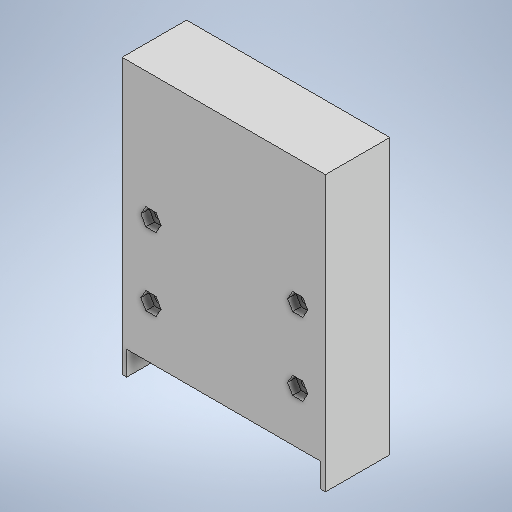
# Autodesk Inventor part: TES_Controller_V1_Case_Top
Saved by Autodesk Inventor 2025 (Build 290162000, 162)
## iProperties
Created: 2025-08-31
Part Number: TES_Controller_V1_Case_Top
Material: 常规
Document SubType Name: Modeling
Designer: 95052
Density: 1 g/cm^3
Appearance: 默认
Author: 95052
Autodesk Inventor part; units mm, degrees
ref_plane "YZ Plane" through (0, 0, 0) normal (1, 0, 0) x (0, 1, 0)
ref_plane "XZ Plane" through (0, 0, 0) normal (0, 1, 0) x (-1, 0, 0)
ref_plane "XY Plane" through (0, 0, 0) normal (0, 0, 1) x (1, 0, 0)
sketch "草图1" plane through (0, 0, 0) normal (0, 0, 1) x (1, 0, 0)
  line L0 (33.589, -45.4) -> (-33.589, -45.4)
  line L1 (-33.589, -45.4) -> (-33.589, 45.4)
  line L2 (-33.589, 45.4) -> (33.589, 45.4)
  line L3 (33.589, 45.4) -> (33.589, -45.4)
  line L4 (33.589, -45.4) -> (-33.589, 45.4) construction
  line L5 (-33.589, -45.4) -> (33.589, 45.4) construction
  line L6 (24.428, -20.313) -> (-24.072, -20.313) construction
  line L7 (-24.072, -20.313) -> (-24.072, 3.687) construction
  line L8 (-24.072, 3.687) -> (24.428, 3.687) construction
  line L9 (24.428, 3.687) -> (24.428, -20.313) construction
  line L10 (-22.3977, 6.587) -> (-20.7234, 3.687)
  line L11 (-20.7234, 3.687) -> (-22.3977, 0.787)
  line L12 (-22.3977, 0.787) -> (-25.7463, 0.787)
  line L13 (-25.7463, 0.787) -> (-27.4206, 3.687)
  line L14 (-27.4206, 3.687) -> (-25.7463, 6.587)
  line L15 (-25.7463, 6.587) -> (-22.3977, 6.587)
  line L16 (-22.3977, -17.413) -> (-20.7234, -20.313)
  line L17 (-20.7234, -20.313) -> (-22.3977, -23.213)
  line L18 (-22.3977, -23.213) -> (-25.7463, -23.213)
  line L19 (-25.7463, -23.213) -> (-27.4206, -20.313)
  line L20 (-27.4206, -20.313) -> (-25.7463, -17.413)
  line L21 (-25.7463, -17.413) -> (-22.3977, -17.413)
  line L22 (26.1023, -17.413) -> (27.7766, -20.313)
  line L23 (27.7766, -20.313) -> (26.1023, -23.213)
  line L24 (26.1023, -23.213) -> (22.7537, -23.213)
  line L25 (22.7537, -23.213) -> (21.0794, -20.313)
  line L26 (21.0794, -20.313) -> (22.7537, -17.413)
  line L27 (22.7537, -17.413) -> (26.1023, -17.413)
  line L28 (22.7537, 0.787) -> (21.0794, 3.687)
  line L29 (21.0794, 3.687) -> (22.7537, 6.587)
  line L30 (22.7537, 6.587) -> (26.1023, 6.587)
  line L31 (26.1023, 6.587) -> (27.7766, 3.687)
  line L32 (27.7766, 3.687) -> (26.1023, 0.787)
  line L33 (26.1023, 0.787) -> (22.7537, 0.787)
  point P0 (0, 0)
  point P1 (-24.072, -17.413)
  point P2 (24.428, -17.413)
  point P3 (24.428, 0.787)
  point P4 (24.428, 6.587)
  dimension "d0" = 90.8
  dimension "d1" = 67.178
  dimension "d2" = 25.087
  dimension "d3" = 9.161
  dimension "d4" = 9.517
  dimension "d5" = 41.713
  dimension "d6" = 2.9
  dimension "d7" = 2.9
  dimension "d8" = 2.9
  dimension "d9" = 2.9
  constraints: 68 end point, 6 midpoint, 4 coincident, 4 parallel, 3 point on line, 2 horizontal, 2 perpendicular, 52 other
  measures "d0" distance of L0.end L1.end
  measures "d1" distance of L0.start L0.end
  measures "d2" distance between parallel lines of L0 L6
  measures "d3" distance between parallel lines of L3 L9
  measures "d4" distance between parallel lines of L1 L7
  measures "d5" distance between parallel lines of L8 L2
  measures "d6" distance from line of L15 L7.end
  measures "d7" distance from line of L21 L6.end
  measures "d8" distance from line of L27 L6.start
  measures "d9" distance of point (24.428, 6.587) L8.end
extrude "拉伸1" add sketch "草图1" along normal blind 2
sketch "草图2" plane through (0, 0, 0) normal (0, 0, -1) x (-1, 0, 0)
  line L0 (22.3977, 0.787) -> (25.7463, 0.787) projected
  line L1 (22.3977, 0.787) -> (20.7234, 3.687)
  line L2 (20.7234, 3.687) -> (22.3977, 6.587)
  line L3 (22.3977, 6.587) -> (25.7463, 6.587)
  line L4 (25.7463, 6.587) -> (27.4206, 3.687)
  line L5 (27.4206, 3.687) -> (25.7463, 0.787)
  line L6 (25.7463, 0.787) -> (22.3977, 0.787)
  line L7 (22.3977, -23.213) -> (25.7463, -23.213) projected
  line L8 (22.3977, -23.213) -> (20.7234, -20.313)
  line L9 (20.7234, -20.313) -> (22.3977, -17.413)
  line L10 (22.3977, -17.413) -> (25.7463, -17.413)
  line L11 (25.7463, -17.413) -> (27.4206, -20.313)
  line L12 (27.4206, -20.313) -> (25.7463, -23.213)
  line L13 (25.7463, -23.213) -> (22.3977, -23.213)
  line L14 (26.3237, 7.587) -> (21.8203, 7.587)
  line L15 (21.8203, 7.587) -> (19.5687, 3.687)
  line L16 (19.5687, 3.687) -> (21.8203, -0.213)
  line L17 (21.8203, -0.213) -> (26.3237, -0.213)
  line L18 (26.3237, -0.213) -> (28.5753, 3.687)
  line L19 (28.5753, 3.687) -> (26.3237, 7.587)
  line L20 (26.3237, -16.413) -> (21.8203, -16.413)
  line L21 (21.8203, -16.413) -> (19.5687, -20.313)
  line L22 (19.5687, -20.313) -> (21.8203, -24.213)
  line L23 (21.8203, -24.213) -> (26.3237, -24.213)
  line L24 (26.3237, -24.213) -> (28.5753, -20.313)
  line L25 (28.5753, -20.313) -> (26.3237, -16.413)
  line L26 (-26.1023, 0.787) -> (-22.7537, 0.787) projected
  line L27 (-26.1023, 0.787) -> (-27.7766, 3.687)
  line L28 (-27.7766, 3.687) -> (-26.1023, 6.587)
  line L29 (-26.1023, 6.587) -> (-22.7537, 6.587)
  line L30 (-22.7537, 6.587) -> (-21.0794, 3.687)
  line L31 (-21.0794, 3.687) -> (-22.7537, 0.787)
  line L32 (-22.7537, 0.787) -> (-26.1023, 0.787)
  line L33 (-22.7537, -17.413) -> (-26.1023, -17.413) projected
  line L34 (-22.7537, -17.413) -> (-21.0794, -20.313)
  line L35 (-21.0794, -20.313) -> (-22.7537, -23.213)
  line L36 (-22.7537, -23.213) -> (-26.1023, -23.213)
  line L37 (-26.1023, -23.213) -> (-27.7766, -20.313)
  line L38 (-27.7766, -20.313) -> (-26.1023, -17.413)
  line L39 (-26.1023, -17.413) -> (-22.7537, -17.413)
  line L40 (-22.1763, -0.213) -> (-19.9247, 3.687)
  line L41 (-19.9247, 3.687) -> (-22.1763, 7.587)
  line L42 (-22.1763, 7.587) -> (-26.6797, 7.587)
  line L43 (-26.6797, 7.587) -> (-28.9313, 3.687)
  line L44 (-28.9313, 3.687) -> (-26.6797, -0.213)
  line L45 (-26.6797, -0.213) -> (-22.1763, -0.213)
  line L46 (-22.1763, -24.213) -> (-19.9247, -20.313)
  line L47 (-19.9247, -20.313) -> (-22.1763, -16.413)
  line L48 (-22.1763, -16.413) -> (-26.6797, -16.413)
  line L49 (-26.6797, -16.413) -> (-28.9313, -20.313)
  line L50 (-28.9313, -20.313) -> (-26.6797, -24.213)
  line L51 (-26.6797, -24.213) -> (-22.1763, -24.213)
  point P0 (0, 0)
  point P1 (24.072, 3.687)
  point P2 (24.072, 0.787)
  point P3 (24.072, -20.313)
  point P4 (24.072, -23.213)
  point P5 (-24.428, 3.687)
  point P6 (-24.428, 0.787)
  point P7 (-24.428, -20.313)
  point P8 (-24.428, -17.413)
  dimension "d13" = 1
  dimension "d14" = 1
  dimension "d24" = 1
  dimension "d25" = 1
  constraints: 96 end point, 8 midpoint, 72 other
  measures "d13" distance between parallel lines of L3 L14
  measures "d14" distance between parallel lines of L10 L20
  measures "d24" distance between parallel lines of L31 L40
  measures "d25" distance between parallel lines of L35 L46
extrude "拉伸2" add sketch "草图2" along normal blind 0.8
sketch "草图4" plane through (0, 0, -0.8) normal (0, 0, -1) x (-1, 0, 0)
  line L0 (19.5687, 3.687) -> (21.8203, -0.213) projected
  line L1 (21.8203, -0.213) -> (19.5687, 3.687)
  line L2 (19.5687, 3.687) -> (21.8203, 7.587)
  line L3 (21.8203, 7.587) -> (26.3237, 7.587)
  line L4 (26.3237, 7.587) -> (28.5753, 3.687)
  line L5 (28.5753, 3.687) -> (26.3237, -0.213)
  line L6 (26.3237, -0.213) -> (21.8203, -0.213)
  line L7 (19.5687, -20.313) -> (21.8203, -16.413) projected
  line L8 (21.8203, -16.413) -> (26.3237, -16.413)
  line L9 (26.3237, -16.413) -> (28.5753, -20.313)
  line L10 (28.5753, -20.313) -> (26.3237, -24.213)
  line L11 (26.3237, -24.213) -> (21.8203, -24.213)
  line L12 (21.8203, -24.213) -> (19.5687, -20.313)
  line L13 (19.5687, -20.313) -> (21.8203, -16.413)
  line L14 (-26.6797, -16.413) -> (-28.9313, -20.313) projected
  line L15 (-26.6797, -16.413) -> (-22.1763, -16.413)
  line L16 (-22.1763, -16.413) -> (-19.9247, -20.313)
  line L17 (-19.9247, -20.313) -> (-22.1763, -24.213)
  line L18 (-22.1763, -24.213) -> (-26.6797, -24.213)
  line L19 (-26.6797, -24.213) -> (-28.9313, -20.313)
  line L20 (-28.9313, -20.313) -> (-26.6797, -16.413)
  line L21 (-26.6797, 7.587) -> (-22.1763, 7.587)
  line L22 (-22.1763, 7.587) -> (-19.9247, 3.687)
  line L23 (-19.9247, 3.687) -> (-22.1763, -0.213)
  line L24 (-22.1763, -0.213) -> (-26.6797, -0.213)
  line L25 (-26.6797, -0.213) -> (-28.9313, 3.687)
  line L26 (-28.9313, 3.687) -> (-26.6797, 7.587)
  circle A0 centre (-24.428, 3.687) radius 1.6
  circle A1 centre (-24.428, -20.313) radius 1.6
  circle A2 centre (24.072, -20.313) radius 1.6
  circle A3 centre (24.072, 3.687) radius 1.6
  point P0 (0, 0)
  dimension "d26" = 3.2
  dimension "d27" = 3.2
  dimension "d28" = 3.2
  dimension "d29" = 3.2
  constraints: 48 end point, 4 centre point, 4 coincident, 52 other
  measures "d26" diameter of A0
  measures "d27" diameter of A1
  measures "d28" diameter of A2
  measures "d29" diameter of A3
extrude "拉伸3" add sketch "草图4" along normal blind 3.5
sketch "草图7" plane through (0, 0, 0) normal (0, 0, -1) x (-1, 0, 0)
  line L0 (33.589, 45.4) -> (33.589, -45.4) projected
  line L1 (33.589, -45.4) -> (-33.589, -45.4) projected
  line L2 (33.589, 45.4) -> (-33.589, 45.4)
  line L3 (-33.589, 45.4) -> (-33.589, -45.4)
  line L4 (33.589, -45.4) -> (33.589, 45.4)
  line L5 (-32.089, 43.9) -> (32.089, 43.9)
  line L6 (32.089, 43.9) -> (32.089, -45.4)
  line L7 (-32.089, -43.9) -> (-32.089, 43.9)
  line L8 (-32.089, -43.9) -> (-32.089, -45.4)
  line L9 (-33.589, -45.4) -> (-32.089, -45.4)
  line L10 (32.089, -45.4) -> (33.589, -45.4)
  point P0 (0, 0)
  dimension "d32" = 1.5
  constraints: 18 end point, 4 parallel, 3 perpendicular, 1 horizontal, 1 other
  measures "d32" distance between parallel lines of L2 L5
extrude "拉伸4" add sketch "草图7" along normal blind 19.3 contours L0 L1 L6 L5 L7 L8 L3 L2
sketch "草图9" plane through (0, 0, 0) normal (0, 0, -1) x (-1, 0, 0)
  line L0 (-32.089, 43.9) -> (-32.089, -45.4) projected
  line L1 (32.089, -45.4) -> (32.089, 43.9) projected
  line L2 (-32.089, -45.4) -> (32.089, -45.4)
  line L3 (32.089, -45.4) -> (32.089, -37.4)
  line L4 (32.089, -37.4) -> (-32.089, -37.4)
  line L5 (-32.089, -37.4) -> (-32.089, -45.4)
  point P0 (0, 0)
  point P1 (-32.089, -37.4)
  dimension "d35" = 8
  constraints: 8 end point, 2 parallel, 1 horizontal, 1 perpendicular, 1 point on line
  measures "d35" distance of L3.end L2.end
extrude "拉伸5" cut sketch "草图9" against normal through all
sketch "草图10" plane through (0, 0, 0) normal (0, 0, -1) x (-1, 0, 0)
  line L0 (-32.089, -37.4) -> (32.089, -37.4) projected
  line L1 (-32.089, 43.9) -> (-32.089, -37.4) projected
  line L2 (32.089, -37.4) -> (-32.089, -37.4)
  line L3 (-32.089, -37.4) -> (-32.089, -35.9)
  line L4 (-32.089, -35.9) -> (32.089, -35.9)
  line L5 (32.089, -35.9) -> (32.089, -37.4)
  point P0 (0, 0)
  dimension "d38" = 1.5
  constraints: 8 end point, 2 parallel, 1 horizontal, 1 perpendicular, 1 point on line
  measures "d38" distance of L2.end L3.end
extrude "拉伸6" add sketch "草图10" along normal blind 11.3
sketch "草图11" plane through (0, 0, -11.3) normal (0, 0, -1) x (-1, 0, 0)
  line L0 (32.089, -37.4) -> (-32.089, -37.4) projected
  line L1 (-32.089, -35.9) -> (32.089, -35.9) projected
  line L2 (20.089, -37.4) -> (-32.089, -37.4)
  line L3 (-32.089, -37.4) -> (-32.089, -35.9)
  line L4 (-32.089, -35.9) -> (20.089, -35.9)
  line L5 (20.089, -35.9) -> (20.089, -37.4)
  line L6 (32.089, 43.9) -> (32.089, -45.4) projected
  line L7 (-32.089, -45.4) -> (-32.089, 43.9) projected
  line L8 (32.089, -35.9) -> (29.289, -35.9)
  line L9 (29.289, -35.9) -> (29.289, -37.4)
  line L10 (29.289, -37.4) -> (32.089, -37.4)
  line L11 (32.089, -37.4) -> (32.089, -35.9)
  point P0 (0, 0)
  point P1 (-32.089, -37.4)
  dimension "d41" = 12
  dimension "d45" = 2.8
  constraints: 16 end point, 4 parallel, 3 point on line, 2 horizontal, 2 perpendicular, 1 collinear
  measures "d41" distance between parallel lines of L6 L5
  measures "d45" distance of L10.end L9.end
extrude "拉伸7" add sketch "草图11" along normal blind 2.5 contours L0 L3 L1 L5
sketch "草图12" plane through (0, 0, -11.3) normal (0, 0, -1) x (-1, 0, 0)
  line L0 (20.089, -37.4) -> (32.089, -37.4) projected
  line L1 (-32.089, -35.9) -> (32.089, -35.9) projected
  line L2 (32.089, -37.4) -> (29.089, -37.4)
  line L3 (29.089, -37.4) -> (29.089, -35.9)
  line L4 (29.089, -35.9) -> (32.089, -35.9)
  line L5 (32.089, -35.9) -> (32.089, -37.4)
  line L6 (-32.089, -35.9) -> (-29.089, -35.9)
  line L7 (-29.089, -35.9) -> (-29.089, -37.4)
  line L8 (-29.089, -37.4) -> (-32.089, -37.4)
  line L9 (-32.089, -37.4) -> (-32.089, -35.9)
  point P0 (0, 0)
  dimension "d46" = 3
  dimension "d47" = 3
  constraints: 16 end point, 4 parallel, 2 horizontal, 2 perpendicular, 2 point on line
  measures "d46" distance of L3.end L4.end
  measures "d47" distance of L7.end L8.end
extrude "拉伸8" add sketch "草图12" along normal up to surface (8 mm away)
